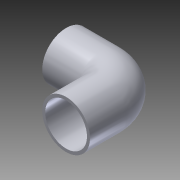
# Autodesk Inventor part: 2 Way Corner
Saved by Autodesk Inventor 2013 (Build 170138000, 138)
## iProperties
Created: 2013-06-24
Part Number: 2 Way Corner
Material: Generic
Document SubType Name: Modeling
Designer: Kyle
Density: 1 g/cm^3
Author: Kyle
Autodesk Inventor part; units mm, degrees
ref_plane "YZ Plane" through (0, 0, 0) normal (1, 0, 0) x (0, 1, 0)
ref_plane "XZ Plane" through (0, 0, 0) normal (0, 1, 0) x (-1, 0, 0)
ref_plane "XY Plane" through (0, 0, 0) normal (0, 0, 1) x (1, 0, 0)
sketch "Sketch1" plane through (0, 0, 0) normal (0, 0, 1) x (1, 0, 0)
  circle A0 centre (0, 0) radius 12.7
  circle A1 centre (0, 0) radius 11.1125
  line L0 (-12.7, 12.7) -> (-12.7, -10.7254)
  line L1 (-12.7, 12.7) -> (16.3739, 12.7)
  dimension "d0" = 25.4
  dimension "d2" = 22.225
  constraints: 4 end point, 2 centre point, 2 tangent, 1 coincident, 1 perpendicular, 1 vertical
  measures "d0" diameter of A0
  measures "d2" diameter of A1
ref_plane "Work Plane1" through (-12.7, 12.7, 0) normal (1, 0, 0) x (0, 1, 0)
sketch "Sketch2" plane through (-12.7, 12.7, 0) normal (1, 0, 0) x (0, 1, 0)
  circle A0 centre (-12.7, -12.7) radius 12.7
  circle A1 centre (-12.7, -12.7) radius 11.1125
  point P0 (-12.7, 0)
  dimension "d3" = 25.4
  dimension "d5" = 12.7
  dimension "d6" = 22.225
  constraints: 2 centre point
  measures "d3" diameter of A0
  measures "d5" distance of point (-12.7, 0) A0.centre
  measures "d6" diameter of A1
extrude "Extrusion1" add sketch "Sketch2" against normal blind 19.05
extrude "Extrusion2" add sketch "Sketch1" along normal blind 19.05 contours A0
sketch "Sketch3" plane through (0, 0, 0) normal (0, 0, -1) x (-1, 0, 0)
  circle A0 centre (0, 0) radius 11.1125 projected
  arc A1 (-12.7, 0) -> (12.7, 0) centre (0, 0) ccw projected
  arc A2 (12.7, 0) -> (-12.7, 0) centre (0, 0) ccw projected
  line L0 (12.7, 14.8538) -> (12.7, -11.8155)
  constraints: 2 end point, 1 tangent, 1 vertical
revolve "Revolution1" add sketch "Sketch3" angle 90 about axis through (-12.7, 14.8538, 0) along (0, 1, 0)
body "Solid1"
